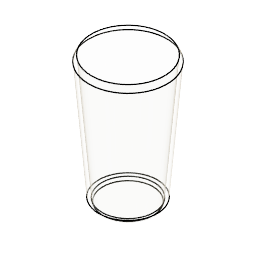
Tapered cup (Autodesk Fusion 360 design; units mm, degrees)
part number: 2026-06-27-13-48-40-281
Autodesk Fusion 360 part; units mm, degrees
sketch "Sketch1" plane through (0, 0, 0) normal (1, 0, 0) x (0, 1, 0)
  line L0 (0, 0) -> (0, 120)
  line L1 (0, 0) -> (27.4, 0)
  line L2 (0, 120) -> (37.5, 120)
  line L3 (37.5, 120) -> (34.5, 120)
  line L4 (27.4, 0) -> (24.4, 0)
  line L5 (27.4, 0) -> (37.5, 120)
  line L6 (34.5, 120) -> (24.4, 0)
  dimension "d1" = 120
  dimension "d2" = 27.4
  dimension "d3" = 37.5
  dimension "d4" = 3
  dimension "d5" = 3
  constraint coincident L0.start L1.start
  constraint vertical L0
  constraint perpendicular L0 L1
  constraint perpendicular L0 L2
  constraint parallel L2 L3
  constraint parallel L1 L4
  measures "d1" distance of L0.start L0.end
  measures "d2" distance of L0.start L1.end
  measures "d3" distance of L0.end L2.end
  measures "d4" distance of L2.end L3.end
  measures "d5" distance of L1.end L4.end
revolve "Revolve1" add sketch "Sketch1" angle 360 about axis through (0, 0, 0) along (0, 0, 1) contours L1 L2 L3 L4 L5 L6
sketch "Sketch2" plane through (0, 0, 0) normal (0, 0, 1) x (1, 0, 0)
  circle A0 centre (0, 0) radius 25
  constraint coincident A0.centre origin
extrude "Extrude1" cut sketch "Sketch2" along normal blind 3
sketch "Sketch3" plane through (0, 0, 0) normal (0, 0, 1) x (1, 0, 0)
sketch "Sketch4" plane through (0, 0, 0) normal (0, 0, 1) x (1, 0, 0)
  circle A0 centre (0, 0) radius 25
  constraint coincident A0.centre origin
extrude "Extrude2" add sketch "Sketch4" along normal blind 3
fillet "Fillet1" radius 6 1 edges at (-34.9623, 13.5606, 120)
fillet "Fillet2" radius 4 1 edges at (-25.5458, 9.9083, 0)
